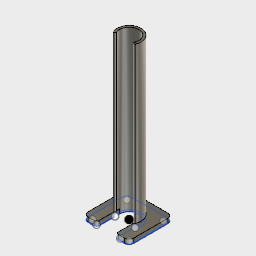
Z-Achse Abstand 70mm v4 (Autodesk Fusion 360 design; units mm, degrees)
Autodesk Fusion 360 part; units mm, degrees
sketch "Skizze1" plane through (0, 0, 0) normal (0, 0, 1) x (1, 0, 0)
  line L0 (8, 9) -> (-8, 9)
  line L1 (-10, 7) -> (-10, -8)
  line L2 (10, -8) -> (10, 7)
  line L3 (-4.25, 0) -> (-4.25, -9)
  line L4 (4.25, 0) -> (4.25, -9)
  line L5 (-4.1679, -2.2229) -> (-4.1679, -2.2229)
  line L6 (4.1679, -2.2229) -> (4.1679, -2.2229)
  arc A0 (3.9397, -1.5942) -> (-3.9397, -1.5942) centre (0, 0) ccw
  arc A1 (4.8667, -1.9692) -> (-4.8667, -1.9692) centre (0, 0) ccw
  line L7 (-8, -10) -> (-5.25, -10)
  line L8 (5.25, -10) -> (8, -10)
  arc A2 (-8, 9) -> (-10, 7) centre (-8, 7) ccw
  arc A3 (10, 7) -> (8, 9) centre (8, 7) ccw
  arc A4 (-10, -8) -> (-8, -10) centre (-8, -8) ccw
  arc A5 (8, -10) -> (10, -8) centre (8, -8) ccw
  arc A6 (-5.25, -10) -> (-4.25, -9) centre (-5.25, -9) ccw
  arc A7 (4.25, -9) -> (5.25, -10) centre (5.25, -9) ccw
  arc A8 (-4.1679, -2.2229) -> (-3.9397, -1.5942) centre (-4.4032, -1.7817) ccw
  arc A9 (-4.8667, -1.9692) -> (-4.1679, -2.2229) centre (-4.4032, -1.7817) ccw
  arc A10 (3.9397, -1.5942) -> (4.1679, -2.2229) centre (4.4032, -1.7817) ccw
  arc A11 (4.1679, -2.2229) -> (4.8667, -1.9692) centre (4.4032, -1.7817) ccw
  dimension "d7" = 2
  dimension "d8" = 2
  dimension "d9" = 2
  dimension "d10" = 2
  dimension "d11" = 1
  dimension "d12" = 1
  dimension "d13" = 0.5
  dimension "d14" = 0.5
  dimension "d15" = 0.5
  dimension "d16" = 0.5
  measures "d7" radius of A2
  measures "d8" radius of A3
  measures "d9" radius of A4
  measures "d10" radius of A5
  measures "d11" radius of A6
  measures "d12" radius of A7
  measures "d13" radius of A8
  measures "d14" radius of A9
  measures "d15" radius of A10
  measures "d16" radius of A11
extrude "Extrusion4" add sketch "Skizze1" along normal blind 2 contours L0 L1 L2 L3 L4 A1 L7 L8 A2 A3 A4 A5 A6 A7 A9 A11 | L3 L4 A0 A1 A9 A11
extrude "Extrusion5" add sketch "Skizze1" along normal blind 70 and the other way blind -2 contours L4 A0 A10 A11 | L3 L4 A0 A1 A9 A11 | L3 A0 A8 A9
equation "d22 = 0.00 °"
